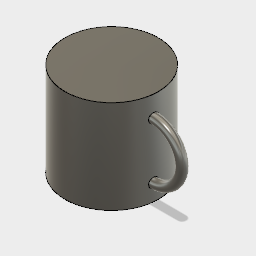
FPROJ_4_Czw (Autodesk Fusion 360 design; units mm, degrees)
Autodesk Fusion 360 part; units mm, degrees
cylinder "圆柱体基本要素1" add diameter 20 height 20 placed x (1, 0, 0) y (0, 0, -1) z (0, 1, 0) at (0, 0, 0) makes body 1
cylinder "圆柱体基本要素2" add diameter 18 height 20 placed x (1, 0, 0) y (0, 0, -1) z (0, 1, 0) at (25, 0, -30) separate body makes body 2
torus "圆环体基本要素1" add centre line diameter 2 section diameter 10 placed x (1, 0, 0) y (0, 0, -1) z (0, 1, 0) at (10, 0, 65) separate body makes body 3
delete_face "删除面1" 1 faces at (7.2967, -2.3627, 69.6822) on bodies 3
torus "圆环体基本要素2" add centre line diameter 12 section diameter 2 placed x (1, 0, 0) y (0, 0, -1) z (0, 1, 0) at (10, 0, 60) separate body makes body 4
move_body "MoveFace1" bodies 4 to x (1, 0, 0) y (0, 1, 0) z (0, 0, 1) at (40, 0, 0) on bodies 4
move_body "MoveFace2" bodies 4 to x (0.996195, 0, 0.087156) y (0, 1, 0) z (-0.087156, 0, 0.996195) at (5.4196, 0, -4.1295) on bodies 4
move_body "MoveFace3" bodies 4 to x (1, 0, 0) y (0, 0, -1) z (0, 1, 0) at (-15, -43.4186, 25.916) on bodies 4
move_body "MoveFace4" bodies 4 to x (1, 0, 0) y (0, 1, 0) z (0, 0, 1) at (-25, 10, -25) on bodies 4
move_body "MoveFace5" bodies 4 to x (1, 0, 0) y (0, 1, 0) z (0, 0, 1) at (0, -20, 0) on bodies 4
move_body "MoveFace6" bodies 4 to x (1, 0, 0) y (0, 1, 0) z (0, 0, 1) at (0, 3, 0) on bodies 4
combine "合并1" operation add target body 1 tool bodies 4
move_body "对齐1" bodies 2 to x (1, 0, 0) y (0, 1, 0) z (0, 0, 1) at (-25, 0, 30)
move_face "偏移面1" offset -2 1 faces at (-5.1676, 20, -0.3267) on bodies 2
combine "合并2" operation cut target body 1 tool bodies 2
